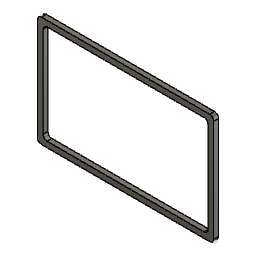
lunette v1 (Autodesk Fusion 360 design; units mm, degrees)
Autodesk Fusion 360 part; units mm, degrees
sketch "Esquisse1" plane through (0, 0, 0) normal (0, 0, 1) x (1, 0, 0)
  line L0 (5, 0) -> (214, 0)
  line L1 (219, 5) -> (219, 132)
  line L2 (214, 137) -> (5, 137)
  line L3 (0, 132) -> (0, 5)
  line L4 (12, 7) -> (207, 7)
  line L5 (212, 12) -> (212, 125)
  line L6 (207, 130) -> (12, 130)
  line L7 (7, 125) -> (7, 12)
  arc A0 (219, 132) -> (214, 137) centre (214, 132) ccw
  arc A1 (212, 125) -> (207, 130) centre (207, 125) ccw
  arc A2 (214, 0) -> (219, 5) centre (214, 5) ccw
  arc A3 (207, 7) -> (212, 12) centre (207, 12) ccw
  arc A4 (7, 12) -> (12, 7) centre (12, 12) ccw
  arc A5 (0, 5) -> (5, 0) centre (5, 5) ccw
  arc A6 (12, 130) -> (7, 125) centre (12, 125) ccw
  arc A7 (5, 137) -> (0, 132) centre (5, 132) ccw
  point P0 (219, 137)
  point P1 (0, 137)
  point P2 (7, 7)
  point P3 (212, 130)
  point P4 (7, 130)
  dimension "d1" = 219
  dimension "d2" = 205
  dimension "d3" = 7
  dimension "d4" = 123
  dimension "d5" = 7
  dimension "d6" = 137
  dimension "d7" = 5
  dimension "d8" = 5
  dimension "d9" = 5
  dimension "d10" = 5
  dimension "d11" = 5
  dimension "d12" = 5
  dimension "d13" = 5
  dimension "d14" = 5
  constraint horizontal L0
  constraint vertical L1
  constraint horizontal L2
  constraint vertical L3
  constraint horizontal L4
  constraint vertical L5
  constraint horizontal L6
  constraint vertical L7
  constraint coincident P0 L1
  constraint coincident P0 L2
  constraint tangent L1 A0
  constraint tangent L2 A0
  constraint coincident P3 L5
  constraint coincident P3 L6
  constraint tangent L5 A1
  constraint tangent L6 A1
  constraint tangent L0 A2
  constraint tangent L1 A2
  constraint tangent L4 A3
  constraint tangent L5 A3
  constraint coincident P2 L4
  constraint coincident P2 L7
  constraint tangent L4 A4
  constraint tangent L7 A4
  constraint coincident origin L0
  constraint coincident origin L3
  constraint tangent L0 A5
  constraint tangent L3 A5
  constraint coincident P4 L6
  constraint coincident P4 L7
  constraint tangent L6 A6
  constraint tangent L7 A6
  constraint coincident P1 L2
  constraint coincident P1 L3
  constraint tangent L2 A7
  constraint tangent L3 A7
  measures "d1" distance of P0 P1
  measures "d2" distance of P3 P4
  measures "d3" distance of L1 L5
  measures "d4" distance of P2 P4
  measures "d5" distance of L0 L4
  measures "d6" distance of origin P1
  measures "d7" radius of A0
  measures "d8" radius of A1
  measures "d9" radius of A2
  measures "d10" radius of A3
  measures "d11" radius of A4
  measures "d12" radius of A5
  measures "d13" radius of A6
  measures "d14" radius of A7
extrude "Extrusion1" add sketch "Esquisse1" along normal blind 6
